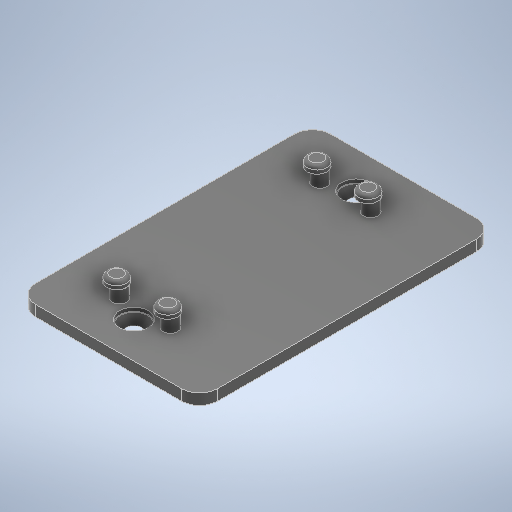
# Autodesk Inventor part: SuportForWall
Saved by Autodesk Inventor 2025 (Build 290162010, 162A)
## iProperties
Created: 2025-11-04
Part Number: SuportForWall
Material: Genérico
Document SubType Name: Modeling
Designer: João Vitor
Density: 1 g/cm^3
Appearance: Suave - Preto
Author: João Vitor
Autodesk Inventor part; units mm, degrees
ref_plane "YZ Plane" through (0, 0, 0) normal (1, 0, 0) x (0, 1, 0)
ref_plane "XZ Plane" through (0, 0, 0) normal (0, 1, 0) x (-1, 0, 0)
ref_plane "XY Plane" through (0, 0, 0) normal (0, 0, 1) x (1, 0, 0)
sketch "Esboço1" plane through (0, 0, 0) normal (0, 1, 0) x (-1, 0, 0)
  line L0 (-20, 37.5) -> (20, 37.5)
  line L1 (22, 35.5) -> (22, -35.5)
  line L2 (20, -37.5) -> (-20, -37.5)
  line L3 (-22, -35.5) -> (-22, 35.5)
  line L4 (-22, 37.5) -> (22, -37.5) construction
  line L5 (22, 37.5) -> (-22, -37.5) construction
  arc A0 (22, 35.5) -> (20, 37.5) centre (20, 35.5) ccw
  arc A1 (-20, 37.5) -> (-22, 35.5) centre (-20, 35.5) ccw
  arc A2 (-22, -35.5) -> (-20, -37.5) centre (-20, -35.5) ccw
  arc A3 (20, -37.5) -> (22, -35.5) centre (20, -35.5) ccw
  line L6 (-20, 40.5) -> (20, 40.5)
  line L7 (25, 35.5) -> (25, -35.5)
  line L8 (20, -40.5) -> (-20, -40.5)
  line L9 (-25, -35.5) -> (-25, 35.5)
  line L10 (-25, 40.5) -> (25, -40.5) construction
  line L11 (25, 40.5) -> (-25, -40.5) construction
  arc A4 (25, 35.5) -> (20, 40.5) centre (20, 35.5) ccw
  arc A5 (20, -40.5) -> (25, -35.5) centre (20, -35.5) ccw
  arc A6 (-25, -35.5) -> (-20, -40.5) centre (-20, -35.5) ccw
  arc A7 (-20, 40.5) -> (-25, 35.5) centre (-20, 35.5) ccw
  point P0 (0, 0)
  dimension "d0" = 75
  dimension "d1" = 44
  dimension "d2" = 2
  dimension "d3" = 3
  dimension "d4" = 3
  dimension "d5" = 5
  constraints: 24 end point, 16 point on circle, 16 point on line, 16 tangent, 8 centre point, 6 equal radius, 4 midpoint, 4 parallel, 2 horizontal, 2 perpendicular
  measures "d0" distance of L5.start L4.end
  measures "d1" distance of L4.end L5.end
  measures "d2" radius of A0
  measures "d3" distance between parallel lines of L7 L1
  measures "d4" distance between parallel lines of L6 L0
  measures "d5" radius of A4
extrude "Extrusão1" add sketch "Esboço1" along normal blind 3 contours L0 A0 L1 A3 L2 A2 L3 A1 | L6 A4 L7 A5 L8 A6 L9 A7
sketch "Esboço2" plane through (0, 3, 0) normal (0, 1, 0) x (1, 0, 0)
  circle A0 centre (-10, -27.5) radius 2
  circle A1 centre (-10, 27.5) radius 2
  circle A2 centre (4, -27.5) radius 2
  circle A3 centre (4, 27.5) radius 2
  line L0 (-20, -40.5) -> (20, -40.5) projected
  line L1 (20, 40.5) -> (-20, 40.5) projected
  point P0 (0, 0)
  dimension "d8" = 4
  dimension "d9" = 13
  dimension "d10" = 4
  dimension "d11" = 10
  dimension "d12" = 13
  constraints: 4 centre point, 3 equal radius, 2 horizontal alignment, 2 vertical alignment
  measures "d8" diameter of A0
  measures "d9" distance from line of L0 A2.centre
  measures "d10" horizontal distance of point (0, 0) A2.centre
  measures "d11" horizontal distance of point (0, 0) A1.centre
  measures "d12" distance from line of A1.centre L1
extrude "Extrusão2" add sketch "Esboço2" along normal blind 3.5
sketch "Esboço3" plane through (-10, 6.5, 27.5) normal (0, 1, 0) x (1, 0, 0)
  circle A0 centre (0, 0) radius 2 projected
  circle A1 centre (14, 0) radius 2 projected
  circle A2 centre (14, 55) radius 2 projected
  circle A3 centre (0, 55) radius 2 projected
  circle A4 centre (-0.75, 0) radius 2.75
  circle A5 centre (0, 0) radius 2 projected
  circle A6 centre (13.25, 0) radius 2.75
  circle A7 centre (13.25, 55) radius 2.75
  circle A8 centre (-0.75, 55) radius 2.75
  circle A9 centre (0, 55) radius 2 projected
  circle A10 centre (14, 55) radius 2 projected
  point P0 (10, 27.5)
  dimension "d15" = 5.5
  constraints: 4 centre point, 4 horizontal alignment, 4 tangent, 3 equal radius
  measures "d15" diameter of A6
extrude "Extrusão3" add sketch "Esboço3" along normal blind 2 contours A0 | A4 | A1 | A6 | A2 | A7 | A3 | A8
fillet "Arredondamento1" radius 1 4 edges at (-13.5, 8.5, -27.5) (0.5, 8.5, -27.5) (-13.5, 8.5, 27.5) (0.5, 8.5, 27.5)
sketch "Esboço4" plane through (0, 3, 0) normal (0, 1, 0) x (1, 0, 0)
  circle A0 centre (-3, -30.5) radius 2.1
  circle A1 centre (-3, 30.5) radius 2.1
  line L0 (-20, -40.5) -> (20, -40.5) projected
  line L1 (20, 40.5) -> (-20, 40.5) projected
  line L2 (-25, 35.5) -> (-25, -35.5) projected
  circle A2 centre (-3, -30.5) radius 4
  circle A3 centre (-3, 30.5) radius 4
  point P0 (0, 0)
  dimension "d19" = 4.2
  dimension "d20" = 10
  dimension "d21" = 10
  dimension "d22" = 22
  dimension "d25" = 8
  constraints: 4 centre point, 2 coincident, 2 equal radius, 1 vertical alignment
  measures "d19" diameter of A1
  measures "d20" distance from line of L0 A0.centre
  measures "d21" distance from line of L1 A1.centre
  measures "d22" distance from line of L2 A1.centre
  measures "d25" diameter of A3
extrude "Extrusão4" cut sketch "Esboço4" against normal blind 10 contours A0 | A1
extrude "Extrusão5" cut sketch "Esboço4" against normal blind 1
sketch "Esboço5" plane through (-3, 2, 30.5) normal (0, 1, 0) x (1, 0, 0)
  circle A0 centre (0, 0) radius 3.75
  circle A1 centre (0, 0) radius 2.1 projected
  circle A2 centre (0, 61) radius 4 projected
  circle A3 centre (0, 61) radius 3.75
  point P0 (3, 30.5)
  dimension "d28" = 7.5
  dimension "d29" = 7.5
  constraints: 2 centre point, 1 coincident, 1 concentric
  measures "d28" diameter of A0
  measures "d29" diameter of A3
chamfer "Chanfro1" distance 2 distance2 1.65 1 edges at (-5.1, 2, 30.5) measured on face at (-0.9068, 0.6667, 30.669)
chamfer "Chanfro2" distance 2 distance2 1.65 1 edges at (-5.1, 2, -30.5) measured on face at (-0.9068, 0.6667, -30.331)
